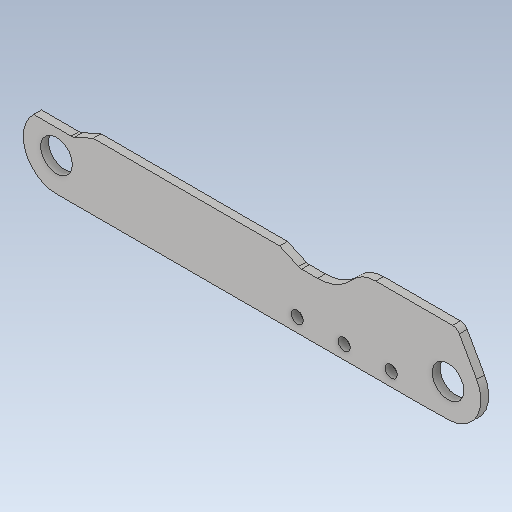
# Autodesk Inventor part: リンク_メインフレーム_6_1
Saved by Autodesk Inventor 2020 (Build 240168000, 168)
## iProperties
Created: 2016-08-23
Part Number: リンク_メインフレーム_6_1
Material: GFRP
Document SubType Name: Modeling
Designer: hiro
Density: 1.75 g/cm^3
Appearance: 滑らか - 淡い灰色
Mass: 6.55334 g
Surface Area: 44.2276 cm^2
Volume: 3.74477 cm^3
Category: リンク
Author: hiro
Autodesk Inventor part; units mm, degrees
ref_plane "YZ Plane" through (0, 0, 0) normal (1, 0, 0) x (0, 1, 0)
ref_plane "XZ Plane" through (0, 0, 0) normal (0, 1, 0) x (-1, 0, 0)
ref_plane "XY Plane" through (0, 0, 0) normal (0, 0, 1) x (1, 0, 0)
sketch "スケッチ1" plane through (0, 0, 0) normal (0, 0, 1) x (1, 0, 0)
  line L0 (-50, 0) -> (50, 0) construction
  circle A0 centre (-50, 0) radius 4.05
  circle A1 centre (50, 0) radius 4.05
  line L1 (-50, 8.5) -> (43, 8.5)
  line L2 (-50, -8.5) -> (43, -8.5)
  arc A2 (-50, 8.5) -> (-50, -8.5) centre (-50, 0) ccw
  line L3 (43, -8.5) -> (50.119, -8.3992)
  line L4 (43, 8.5) -> (50.119, 8.3992)
  arc A3 (50.119, -8.3992) -> (50.119, 8.3992) centre (50, 0) ccw
  line L5 (9, -7.5) -> (38, -7.5) construction
  line L6 (38, -7.5) -> (38, -2.5) construction
  line L7 (38, -2.5) -> (9, -2.5) construction
  line L8 (9, -2.5) -> (9, -7.5) construction
  line L9 (9, -5) -> (38, -5) construction
  circle A4 centre (23.5, -5) radius 1.55
  circle A5 centre (11.5, -5) radius 1.55
  circle A6 centre (35.5, -5) radius 1.55
  line L10 (23.5, -5) -> (23.5, -2.5) construction
  line L11 (52.3191, 13) -> (22.3191, 13)
  line L12 (22.3191, 13) -> (12.3191, 8.5)
  line L13 (52.3191, 13) -> (57.3191, 4.122)
  point P0 (0, 0)
  point P1 (0, 0)
  point P2 (54.8534, 8.5)
  dimension "d0" = 100
  dimension "d1" = 8.1
  dimension "d2" = 8.5
  dimension "d8" = 8.1
  dimension "d9" = 7
  dimension "d10" = 8.4
  dimension "d12" = 5
  dimension "d13" = 29
  dimension "d14" = 3.1
  dimension "d15" = 2.5
  dimension "d17" = 13
  dimension "d19" = 10
  dimension "d20" = 30
  dimension "d25" = 12
  dimension "d26" = 5
  dimension "d45" = 1
  constraints: 28 end point, 7 centre point, 5 horizontal, 5 midpoint, 5 point on circle, 5 point on line, 5 tangent, 4 coincident, 2 equal radius, 2 parallel, 1 perpendicular, 1 symmetric about line, 1 vertical alignment
  measures "d0" distance of L0.start L0.end
  measures "d1" diameter of A0
  measures "d2" radius of A2
  measures "d8" diameter of A1
  measures "d9" horizontal distance of L1.end L0.end
  measures "d10" radius of A3
  measures "d12" distance of L7.end L5.start
  measures "d13" distance of L6.end L7.end
  measures "d14" diameter of A4
  measures "d15" distance from line of L8 A5.centre
  measures "d17" distance from line of L0.end L11
  measures "d19" horizontal distance of L12.end L11.end
  measures "d20" distance of L11.start L11.end
  measures "d25" distance from line of L0.end L6
  measures "d26" horizontal distance of L11.start L13.end
  measures "d45" distance between parallel lines of L2 L5
extrude "押し出し1" add sketch "スケッチ1" along normal blind 2
fillet "フィレット1" radius 2 3 edges at (12.3191, 8.5, 1) (22.3191, 13, 1) (52.3191, 13, 1)
sketch "スケッチ2" plane through (0, 0, 0) normal (0, 0, -1) x (-1, 0, 0)
  circle A0 centre (-16.6795, 17.7128) radius 11.35 construction
  circle A1 centre (-16.6795, 17.7128) radius 11.55
  line L0 (-16.6795, 6.1628) -> (58.7547, 6.1628)
  line L1 (-16.6795, 17.7128) -> (-34, 27.7128) construction
  circle A2 centre (-50, 0) radius 4.05 projected
  line L2 (-50, 0) -> (-34, 27.7128) construction
  line L3 (50, -8.5) -> (-43, -8.5) projected
  line L4 (-2.1795, 10.6628) -> (35.8205, 10.6628)
  line L5 (35.8205, 10.6628) -> (45.8205, 6.1628)
  line L6 (-2.1795, 10.6628) -> (-12.1795, 6.1628)
  circle A3 centre (50, 0) radius 4.05 projected
  line L7 (58.7547, 6.1628) -> (-13.2236, 28.7337)
  arc A4 (50, -8.5) -> (50, 8.5) centre (50, 0) ccw projected
  point P0 (0, 0)
  dimension "d29" = 22.7
  dimension "d30" = 0.2
  dimension "d31" = 60
  dimension "d32" = 90
  dimension "d33" = 20
  dimension "d34" = 38
  dimension "d35" = 10
  dimension "d36" = 10
  dimension "d37" = 4.5
  dimension "d38" = 32
  dimension "d40" = 4.5
  constraints: 14 end point, 3 tangent, 2 centre point, 2 horizontal, 2 point on circle, 2 point on line
  measures "d29" diameter of A0
  measures "d30" radial gap between concentric circles of A0 A1
  measures "d31" angle of L3 L2
  measures "d32" angle of L1 L2
  measures "d33" distance from line of L1.start L2
  measures "d34" distance of L4.start L4.end
  measures "d35" horizontal distance of L4.start L6.end
  measures "d36" horizontal distance of L5.end L4.end
  measures "d37" distance between parallel lines of L0 L4
  measures "d38" distance from line of L2.start L1
  measures "d40" horizontal distance of L6.end L1.start
extrude "押し出し2" cut sketch "スケッチ2" against normal through all contours A1 | A1 L7 A4 L0 L5 L4 L6 | L7 L0 A4
fillet "フィレット2" radius 8 1 edges at (27.2242, 13, 1)
fillet "フィレット2" radius 2 2 edges at (12.1795, 6.1628, 1) (-45.8205, 6.1628, 1)
equation "\"d8\" = d1"
equation "\"d19\" = d18"
equation "\"d36\" = d35"
equation "\"d18\" = 10"
